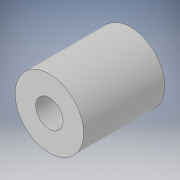
# Autodesk Inventor part: Acople eje motor
Saved by Autodesk Inventor 2019 (Build 230136000, 136)
## iProperties
Created: 2020-02-01
Part Number: Acople eje motor
Material: Generic
Document SubType Name: Modeling
Designer: Elías Sánchez
Density: 1 g/cm^3
Appearance: Default
Author: Elías Sánchez
Autodesk Inventor part; units mm, degrees
ref_plane "YZ Plane" through (0, 0, 0) normal (1, 0, 0) x (0, 1, 0)
ref_plane "XZ Plane" through (0, 0, 0) normal (0, 1, 0) x (-1, 0, 0)
sketch "Sketch1" plane through (0, 0, 0) normal (0, 0, 1) x (1, 0, 0)
  circle A0 centre (0, 0) radius 7.5
  circle A1 centre (0, 0) radius 3
  dimension "d0" = 15
  dimension "d1" = 6
  constraints: 2 centre point, 2 coincident
  measures "d0" diameter of A0
  measures "d1" diameter of A1
extrude "Extrusion1" add sketch "Sketch1" along normal blind 17.8
ref_plane "Work Plane1" through (0, 0, 5) normal (0, 0, 1) x (1, 0, 0)
sketch "Sketch2" plane through (0, 0, 5) normal (0, 0, 1) x (1, 0, 0)
  line L0 (-5.5, -2.6) -> (-3.3, -2.6)
  line L1 (-3.3, -2.6) -> (-3.3, 2.6)
  line L2 (-3.3, 2.6) -> (-5.5, 2.6)
  line L3 (-5.5, 2.6) -> (-5.5, -2.6)
  point P0 (0, 0)
  point P1 (-5.5, 0)
  dimension "d5" = 5.5
  dimension "d6" = 2.2
  dimension "d7" = 5.2
  constraints: 8 end point, 2 parallel, 1 horizontal, 1 horizontal alignment, 1 midpoint, 1 perpendicular
  measures "d5" distance from line of point (0, 0) L3
  measures "d6" distance between parallel lines of L1 L3
  measures "d7" distance of L2.end L0.start
extrude "Extrusion2" cut sketch "Sketch2" along normal mid plane 10
sketch "Sketch4" plane through (0, 0, 0) normal (1, 0, 0) x (0, 1, 0)
  circle A0 centre (0, 4) radius 1.5
  line L0 (-2.1, 0) -> (2.1, 0) projected
  point P0 (0, 0)
  dimension "d12" = 3
  dimension "d13" = 4
  constraints: 1 centre point, 1 vertical alignment
  measures "d12" diameter of A0
  measures "d13" distance from line of L0 A0.centre
extrude "Extrusion3" cut sketch "Sketch4" against normal blind 8
sketch "Sketch5" plane through (0, 0, 0) normal (0, 1, 0) x (-1, 0, 0)
  line L0 (7.5, 0) -> (7.5, 17.8) projected
  line L1 (7.5, 1) -> (7, 1)
  line L2 (7, 1) -> (7, 7)
  line L3 (7, 7) -> (7.5, 7)
  line L4 (7.5, 7) -> (7.5, 1)
  line L5 (-1.5, 0) -> (9, 0) projected
  point P0 (0, 0)
  dimension "d16" = 6
  dimension "d17" = 7
  dimension "d18" = 0.5
  constraints: 8 end point, 2 parallel, 1 horizontal, 1 perpendicular, 1 point on line
  measures "d16" distance of L1.end L2.end
  measures "d17" distance between parallel lines of L5 L3
  measures "d18" distance between parallel lines of L2 L0
extrude "Extrusion4" cut sketch "Sketch5" along normal mid plane 8
body "Solid1"
